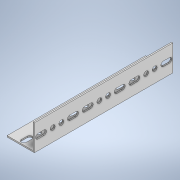
# Autodesk Inventor part: ChassisFrame
Saved by Autodesk Inventor 2020 (Build 240168000, 168)
## iProperties
Created: 2021-11-11
Part Number: ChassisFrame
Material: Generic
Document SubType Name: Modeling
Designer: 17185
Density: 1 g/cm^3
Appearance: Default
Author: 17185
Autodesk Inventor part; units mm, degrees
ref_plane "YZ Plane" through (0, 0, 0) normal (1, 0, 0) x (0, 1, 0)
ref_plane "XZ Plane" through (0, 0, 0) normal (0, 1, 0) x (-1, 0, 0)
ref_plane "XY Plane" through (0, 0, 0) normal (0, 0, 1) x (1, 0, 0)
sketch "Sketch1" plane through (0, 0, 0) normal (0, 1, 0) x (-1, 0, 0)
  line L0 (19.05, 101.6) -> (-19.05, 101.6)
  line L1 (-19.05, 101.6) -> (-19.05, -101.6)
  line L2 (-19.05, -101.6) -> (19.05, -101.6)
  line L3 (19.05, -101.6) -> (19.05, 101.6)
  line L4 (19.05, 101.6) -> (-19.05, -101.6) construction
  line L5 (-19.05, 101.6) -> (19.05, -101.6) construction
  circle A0 centre (0, 62.23) radius 3.556
  circle A1 centre (0, 6.35) radius 3.556
  line L6 (0, 101.6) -> (0, -101.6) construction
  line L7 (0, 49.53) -> (0, 40.64) construction
  line L8 (3.556, 49.53) -> (3.556, 40.64)
  line L9 (-3.556, 40.64) -> (-3.556, 49.53)
  arc A2 (3.556, 49.53) -> (-3.556, 49.53) centre (0, 49.53) ccw
  arc A3 (-3.556, 40.64) -> (3.556, 40.64) centre (0, 40.64) ccw
  line L10 (0, 27.94) -> (0, 19.05) construction
  line L11 (-3.556, 27.94) -> (-3.556, 19.05)
  line L12 (3.556, 19.05) -> (3.556, 27.94)
  arc A4 (3.556, 27.94) -> (-3.556, 27.94) centre (0, 27.94) ccw
  arc A5 (-3.556, 19.05) -> (3.556, 19.05) centre (0, 19.05) ccw
  line L13 (19.05, 68.58) -> (-6.1251, 68.58) construction
  line L14 (-6.1251, 68.58) -> (-19.05, 68.58) construction
  circle A6 centre (0, 74.93) radius 3.556
  circle A7 centre (0, 130.81) radius 3.556
  line L15 (0, 87.63) -> (0, 96.52) construction
  line L16 (3.556, 87.63) -> (3.556, 96.52)
  line L17 (-3.556, 96.52) -> (-3.556, 87.63)
  arc A8 (-3.556, 87.63) -> (3.556, 87.63) centre (0, 87.63) ccw
  arc A9 (3.556, 96.52) -> (-3.556, 96.52) centre (0, 96.52) ccw
  line L18 (0, 109.22) -> (0, 118.11) construction
  line L19 (-3.556, 109.22) -> (-3.556, 118.11)
  line L20 (3.556, 118.11) -> (3.556, 109.22)
  arc A10 (-3.556, 109.22) -> (3.556, 109.22) centre (0, 109.22) ccw
  arc A11 (3.556, 118.11) -> (-3.556, 118.11) centre (0, 118.11) ccw
  line L21 (19.05, 0) -> (-19.05, 0) construction
  circle A12 centre (0, -62.23) radius 3.556
  circle A13 centre (0, -6.35) radius 3.556
  line L22 (0, -49.53) -> (0, -40.64) construction
  line L23 (3.556, -49.53) -> (3.556, -40.64)
  line L24 (-3.556, -40.64) -> (-3.556, -49.53)
  arc A14 (-3.556, -49.53) -> (3.556, -49.53) centre (0, -49.53) ccw
  arc A15 (3.556, -40.64) -> (-3.556, -40.64) centre (0, -40.64) ccw
  line L25 (0, -27.94) -> (0, -19.05) construction
  line L26 (-3.556, -27.94) -> (-3.556, -19.05)
  line L27 (3.556, -19.05) -> (3.556, -27.94)
  arc A16 (-3.556, -27.94) -> (3.556, -27.94) centre (0, -27.94) ccw
  arc A17 (3.556, -19.05) -> (-3.556, -19.05) centre (0, -19.05) ccw
  line L28 (0, -109.22) -> (0, -118.11) construction
  line L29 (3.556, -118.11) -> (3.556, -109.22)
  arc A18 (3.556, -109.22) -> (-3.556, -109.22) centre (0, -109.22) ccw
  arc A19 (-3.556, -118.11) -> (3.556, -118.11) centre (0, -118.11) ccw
  circle A20 centre (0, -130.81) radius 3.556
  line L30 (-3.556, -109.22) -> (-3.556, -118.11)
  line L31 (0, -87.63) -> (0, -96.52) construction
  line L32 (-3.556, -96.52) -> (-3.556, -87.63)
  arc A21 (-3.556, -96.52) -> (3.556, -96.52) centre (0, -96.52) ccw
  arc A22 (3.556, -87.63) -> (-3.556, -87.63) centre (0, -87.63) ccw
  circle A23 centre (0, -74.93) radius 3.556
  line L33 (3.556, -87.63) -> (3.556, -96.52)
  line L34 (19.05, -137.16) -> (-19.05, -137.16) construction
  line L35 (19.05, 137.16) -> (-19.05, 137.16) construction
  circle A24 centre (0, 212.09) radius 3.556
  circle A25 centre (0, 267.97) radius 3.556
  line L36 (0, 224.79) -> (0, 233.68) construction
  line L37 (3.556, 224.79) -> (3.556, 233.68)
  line L38 (-3.556, 233.68) -> (-3.556, 224.79)
  arc A26 (-3.556, 224.79) -> (3.556, 224.79) centre (0, 224.79) ccw
  arc A27 (3.556, 233.68) -> (-3.556, 233.68) centre (0, 233.68) ccw
  line L39 (0, 246.38) -> (0, 255.27) construction
  line L40 (-3.556, 246.38) -> (-3.556, 255.27)
  line L41 (3.556, 255.27) -> (3.556, 246.38)
  arc A28 (-3.556, 246.38) -> (3.556, 246.38) centre (0, 246.38) ccw
  arc A29 (3.556, 255.27) -> (-3.556, 255.27) centre (0, 255.27) ccw
  line L42 (0, 165.1) -> (0, 156.21) construction
  line L43 (3.556, 156.21) -> (3.556, 165.1)
  arc A30 (3.556, 165.1) -> (-3.556, 165.1) centre (0, 165.1) ccw
  arc A31 (-3.556, 156.21) -> (3.556, 156.21) centre (0, 156.21) ccw
  circle A32 centre (0, 143.51) radius 3.556
  line L44 (-3.556, 165.1) -> (-3.556, 156.21)
  line L45 (0, 186.69) -> (0, 177.8) construction
  line L46 (-3.556, 177.8) -> (-3.556, 186.69)
  arc A33 (-3.556, 177.8) -> (3.556, 177.8) centre (0, 177.8) ccw
  arc A34 (3.556, 186.69) -> (-3.556, 186.69) centre (0, 186.69) ccw
  circle A35 centre (0, 199.39) radius 3.556
  line L47 (3.556, 186.69) -> (3.556, 177.8)
  arc A36 (3.556, 302.26) -> (-3.556, 302.26) centre (0, 302.26) ccw
  arc A37 (-3.556, 293.37) -> (3.556, 293.37) centre (0, 293.37) ccw
  circle A38 centre (0, 280.67) radius 3.556
  line L48 (-3.556, 302.26) -> (-3.556, 293.37)
  line L49 (3.556, 293.37) -> (3.556, 302.26)
  line L50 (0, 302.26) -> (0, 293.37) construction
  circle A39 centre (0, -280.67) radius 3.556
  line L51 (0, -302.26) -> (0, -293.37) construction
  line L52 (-3.556, -302.26) -> (-3.556, -293.37)
  line L53 (3.556, -293.37) -> (3.556, -302.26)
  arc A40 (-3.556, -302.26) -> (3.556, -302.26) centre (0, -302.26) ccw
  arc A41 (3.556, -293.37) -> (-3.556, -293.37) centre (0, -293.37) ccw
  line L54 (19.05, -274.32) -> (-19.05, -274.32) construction
  arc A42 (3.556, -246.38) -> (-3.556, -246.38) centre (0, -246.38) ccw
  arc A43 (-3.556, -255.27) -> (3.556, -255.27) centre (0, -255.27) ccw
  circle A44 centre (0, -267.97) radius 3.556
  line L55 (-3.556, -246.38) -> (-3.556, -255.27)
  line L56 (3.556, -255.27) -> (3.556, -246.38)
  line L57 (0, -246.38) -> (0, -255.27) construction
  line L58 (0, -224.79) -> (0, -233.68) construction
  line L59 (-3.556, -233.68) -> (-3.556, -224.79)
  circle A45 centre (0, -212.09) radius 3.556
  arc A46 (3.556, -224.79) -> (-3.556, -224.79) centre (0, -224.79) ccw
  line L60 (3.556, -224.79) -> (3.556, -233.68)
  arc A47 (-3.556, -233.68) -> (3.556, -233.68) centre (0, -233.68) ccw
  arc A48 (3.556, -177.8) -> (-3.556, -177.8) centre (0, -177.8) ccw
  arc A49 (-3.556, -165.1) -> (3.556, -165.1) centre (0, -165.1) ccw
  line L61 (0, -165.1) -> (0, -156.21) construction
  line L62 (-3.556, -165.1) -> (-3.556, -156.21)
  line L63 (3.556, -156.21) -> (3.556, -165.1)
  arc A50 (3.556, -156.21) -> (-3.556, -156.21) centre (0, -156.21) ccw
  circle A51 centre (0, -143.51) radius 3.556
  line L64 (0, -186.69) -> (0, -177.8) construction
  line L65 (-3.556, -177.8) -> (-3.556, -186.69)
  line L66 (3.556, -186.69) -> (3.556, -177.8)
  arc A52 (-3.556, -186.69) -> (3.556, -186.69) centre (0, -186.69) ccw
  circle A53 centre (0, -199.39) radius 3.556
  point P0 (0, 0)
  point P1 (0, 45.085)
  point P2 (0, 23.495)
  point P3 (0, 92.075)
  point P4 (0, 113.665)
  point P5 (0, -45.085)
  point P6 (0, -23.495)
  point P7 (-6.1251, -68.58)
  point P8 (0, -113.665)
  point P9 (0, -92.075)
  point P10 (0, 274.32)
  point P11 (0, 229.235)
  point P12 (0, 250.825)
  point P13 (-6.1251, 205.74)
  point P14 (0, 160.655)
  point P15 (0, 182.245)
  point P16 (0, 297.815)
  point P17 (0, -274.32)
  point P18 (0, -297.815)
  point P19 (0, -250.825)
  point P20 (0, -229.235)
  point P21 (0, -160.655)
  point P22 (-6.1251, -205.74)
  point P23 (0, -182.245)
  point P24 (2.4887, -304.8)
  point P25 (2.4887, 304.8)
  point P26 (-2.4887, 304.8)
  point P27 (-2.4887, -304.8)
  dimension "d1" = 203.2
  dimension "d3" = 7.112
  dimension "d6" = 7.112
  dimension "d9" = 3.556
  dimension "d10" = 3.556
  dimension "d11" = 6.35
  dimension "d12" = 12.7
  dimension "d13" = 8.89
  dimension "d14" = 8.89
  dimension "d15" = 12.7
  dimension "d16" = 12.7
  dimension "d26" = 6.35
  dimension "d29" = 6.35
  dimension "d30" = 6.35
  constraints: 170 end point, 135 symmetric about line, 72 point on circle, 54 centre point, 11 point on line, 8 midpoint, 8 tangent, 4 parallel, 3 perpendicular, 2 horizontal, 48 other
  measures "d1" distance of L0.end L1.end
  measures "d3" diameter of A1
  measures "d6" diameter of A0
  measures "d9" radius of A5
  measures "d10" radius of A3
  measures "d11" distance of A1.centre point (0, 0)
  measures "d12" distance of L10.end A1.centre
  measures "d13" distance of L10.start L10.end
  measures "d14" distance of L7.start L7.end
  measures "d15" distance of L10.start L7.end
  measures "d16" distance of L7.start A0.centre
  measures "d26" distance from line of A0.centre L13
  measures "d29" distance from line of L34 A20.centre
  measures "d30" distance from line of L35 A7.centre
extrude "Extrusion1" add sketch "Sketch1" along normal blind 1.9844 contours L3 L2 L1 L0
sketch "Sketch5" plane through (19.05, 0, 101.6) normal (1, 0, 0) x (0, 0, -1)
  line L0 (0.0028, 0.1675) -> (203.2028, 0.1675)
  line L1 (203.2028, 0.1675) -> (203.2028, 38.2675)
  line L2 (203.2028, 38.2675) -> (0.0028, 38.2675)
  line L3 (0.0028, 38.2675) -> (0.0028, 0.1675)
  line L4 (101.6, 0) -> (101.6028, 38.2675) construction
  line L5 (0.0028, 18.2829) -> (203.2028, 19.2175) construction
  circle A0 centre (95.2514, 18.721) radius 3.556
  line L6 (82.5514, 18.6626) -> (73.6615, 18.6217) construction
  line L7 (82.535, 22.2186) -> (73.6451, 22.1777)
  line L8 (73.6778, 15.0658) -> (82.5677, 15.1066)
  arc A1 (82.5677, 15.1066) -> (82.535, 22.2186) centre (82.5514, 18.6626) ccw
  arc A2 (73.6451, 22.1777) -> (73.6778, 15.0658) centre (73.6615, 18.6217) ccw
  line L9 (0, 0) -> (203.2, 0) construction
  line L10 (67.3115, 38.2675) -> (67.3115, 0) construction
  circle A3 centre (39.3716, 18.721) radius 3.556
  line L11 (52.0716, 18.6626) -> (60.9615, 18.6217) construction
  line L12 (52.0879, 22.2186) -> (60.9778, 22.1777)
  line L13 (60.9451, 15.0658) -> (52.0552, 15.1066)
  arc A4 (52.0879, 22.2186) -> (52.0552, 15.1066) centre (52.0716, 18.6626) ccw
  arc A5 (60.9451, 15.0658) -> (60.9778, 22.1777) centre (60.9615, 18.6217) ccw
  line L14 (33.0216, 38.2675) -> (33.0216, 0) construction
  circle A6 centre (-29.2082, 18.721) radius 3.556
  line L15 (-16.5082, 18.6626) -> (-7.6183, 18.6217) construction
  line L16 (-16.4919, 22.2186) -> (-7.602, 22.1777)
  line L17 (-7.6347, 15.0658) -> (-16.5246, 15.1066)
  arc A7 (-16.4919, 22.2186) -> (-16.5246, 15.1066) centre (-16.5082, 18.6626) ccw
  arc A8 (-7.6347, 15.0658) -> (-7.602, 22.1777) centre (-7.6183, 18.6217) ccw
  line L18 (13.9716, 18.6626) -> (5.0817, 18.6217) construction
  line L19 (5.098, 15.0658) -> (13.9879, 15.1066)
  arc A9 (5.0653, 22.1777) -> (5.098, 15.0658) centre (5.0817, 18.6217) ccw
  circle A10 centre (26.6716, 18.721) radius 3.556
  arc A11 (13.9879, 15.1066) -> (13.9552, 22.2186) centre (13.9716, 18.6626) ccw
  line L20 (13.9552, 22.2186) -> (5.0653, 22.1777)
  line L21 (-35.5582, 38.2675) -> (-35.5582, 0) construction
  circle A12 centre (-166.3679, 18.721) radius 3.556
  line L22 (-153.6679, 18.6626) -> (-144.778, 18.6217) construction
  line L23 (-153.6515, 22.2186) -> (-144.7616, 22.1777)
  line L24 (-144.7943, 15.0658) -> (-153.6842, 15.1066)
  arc A13 (-153.6515, 22.2186) -> (-153.6842, 15.1066) centre (-153.6679, 18.6626) ccw
  arc A14 (-144.7943, 15.0658) -> (-144.7616, 22.1777) centre (-144.778, 18.6217) ccw
  line L25 (-123.188, 18.6626) -> (-132.078, 18.6217) construction
  line L26 (-132.0616, 15.0658) -> (-123.1717, 15.1066)
  arc A15 (-132.0943, 22.1777) -> (-132.0616, 15.0658) centre (-132.078, 18.6217) ccw
  circle A16 centre (-110.488, 18.721) radius 3.556
  arc A17 (-123.1717, 15.1066) -> (-123.2044, 22.2186) centre (-123.188, 18.6626) ccw
  line L27 (-123.2044, 22.2186) -> (-132.0943, 22.1777)
  arc A18 (-85.0717, 22.2186) -> (-85.1044, 15.1066) centre (-85.088, 18.6626) ccw
  line L28 (-85.088, 18.6626) -> (-76.1981, 18.6217) construction
  line L29 (-85.0717, 22.2186) -> (-76.1818, 22.1777)
  arc A19 (-76.2145, 15.0658) -> (-76.1818, 22.1777) centre (-76.1981, 18.6217) ccw
  arc A20 (-63.5145, 22.1777) -> (-63.4818, 15.0658) centre (-63.4981, 18.6217) ccw
  line L30 (-54.6246, 22.2186) -> (-63.5145, 22.1777)
  line L31 (-63.4818, 15.0658) -> (-54.5919, 15.1066)
  arc A21 (-54.5919, 15.1066) -> (-54.6246, 22.2186) centre (-54.6082, 18.6626) ccw
  circle A22 centre (-41.9082, 18.721) radius 3.556
  circle A23 centre (-97.788, 18.721) radius 3.556
  line L32 (-54.6082, 18.6626) -> (-63.4981, 18.6217) construction
  line L33 (-76.2145, 15.0658) -> (-85.1044, 15.1066)
  line L34 (-172.7179, 38.2675) -> (-172.7179, 0) construction
  arc A24 (-191.7515, 15.1066) -> (-191.7842, 22.2186) centre (-191.7679, 18.6626) ccw
  line L35 (-191.7679, 18.6626) -> (-200.6578, 18.6217) construction
  line L36 (-200.6414, 15.0658) -> (-191.7515, 15.1066)
  arc A25 (-200.6741, 22.1777) -> (-200.6414, 15.0658) centre (-200.6578, 18.6217) ccw
  circle A26 centre (-179.0679, 18.721) radius 3.556
  line L37 (-191.7842, 22.2186) -> (-200.6741, 22.1777)
  circle A27 centre (107.9514, 18.7201) radius 3.556
  line L38 (120.6514, 18.6598) -> (129.5413, 18.6176) construction
  line L39 (120.6683, 22.2157) -> (129.5582, 22.1735)
  line L40 (129.5244, 15.0616) -> (120.6345, 15.1038)
  arc A28 (120.6683, 22.2157) -> (120.6345, 15.1038) centre (120.6514, 18.6598) ccw
  arc A29 (129.5244, 15.0616) -> (129.5582, 22.1735) centre (129.5413, 18.6176) ccw
  line L41 (151.1312, 18.6553) -> (142.2413, 18.6157) construction
  line L42 (142.2571, 15.0597) -> (151.147, 15.0993)
  arc A30 (142.2255, 22.1717) -> (142.2571, 15.0597) centre (142.2413, 18.6157) ccw
  circle A31 centre (163.8312, 18.7118) radius 3.556
  arc A32 (151.147, 15.0993) -> (151.1154, 22.2112) centre (151.1312, 18.6553) ccw
  line L43 (151.1154, 22.2112) -> (142.2255, 22.1717)
  arc A33 (189.2481, 22.2056) -> (189.2143, 15.0936) centre (189.2312, 18.6496) ccw
  line L44 (189.2312, 18.6496) -> (198.1211, 18.6074) construction
  line L45 (189.2481, 22.2056) -> (198.138, 22.1634)
  arc A34 (198.1042, 15.0514) -> (198.138, 22.1634) centre (198.1211, 18.6074) ccw
  arc A35 (210.8053, 22.1615) -> (210.8369, 15.0496) centre (210.8211, 18.6055) ccw
  line L46 (219.6952, 22.2011) -> (210.8053, 22.1615)
  line L47 (210.8369, 15.0496) -> (219.7268, 15.0891)
  arc A36 (219.7268, 15.0891) -> (219.6952, 22.2011) centre (219.711, 18.6451) ccw
  circle A37 centre (232.411, 18.7016) radius 3.556
  circle A38 centre (176.5312, 18.7099) radius 3.556
  line L48 (219.711, 18.6451) -> (210.8211, 18.6055) construction
  line L49 (198.1042, 15.0514) -> (189.2143, 15.0936)
  arc A39 (356.8865, 15.0688) -> (356.8548, 22.1807) centre (356.8706, 18.6247) ccw
  line L50 (356.8706, 18.6247) -> (347.9807, 18.5852) construction
  line L51 (347.9965, 15.0292) -> (356.8865, 15.0688)
  arc A40 (347.9649, 22.1411) -> (347.9965, 15.0292) centre (347.9807, 18.5852) ccw
  arc A41 (335.2638, 15.0311) -> (335.2976, 22.143) centre (335.2807, 18.5871) ccw
  line L52 (326.3908, 18.6293) -> (335.2807, 18.5871) construction
  arc A42 (326.4077, 22.1852) -> (326.3739, 15.0733) centre (326.3908, 18.6293) ccw
  circle A43 centre (369.5706, 18.6813) radius 3.556
  line L53 (356.8548, 22.1807) -> (347.9649, 22.1411)
  circle A44 centre (313.6908, 18.6896) radius 3.556
  line L54 (326.4077, 22.1852) -> (335.2976, 22.143)
  line L55 (335.2638, 15.0311) -> (326.3739, 15.0733)
  circle A45 centre (300.9908, 18.6914) radius 3.556
  arc A46 (288.3066, 15.079) -> (288.275, 22.1909) centre (288.2908, 18.6349) ccw
  line L56 (288.275, 22.1909) -> (279.3851, 22.1513)
  line L57 (288.2908, 18.6349) -> (279.4009, 18.5953) construction
  line L58 (279.4167, 15.0394) -> (288.3066, 15.079)
  arc A47 (279.3851, 22.1513) -> (279.4167, 15.0394) centre (279.4009, 18.5953) ccw
  arc A48 (266.684, 15.0413) -> (266.7178, 22.1532) centre (266.7009, 18.5972) ccw
  line L59 (257.8279, 22.1954) -> (266.7178, 22.1532)
  line L60 (257.811, 18.6394) -> (266.7009, 18.5972) construction
  line L61 (266.684, 15.0413) -> (257.7941, 15.0835)
  arc A49 (257.8279, 22.1954) -> (257.7941, 15.0835) centre (257.811, 18.6394) ccw
  circle A50 centre (245.111, 18.6997) radius 3.556
  arc A51 (394.9875, 22.1751) -> (394.9537, 15.0631) centre (394.9706, 18.6191) ccw
  line L62 (394.9706, 18.6191) -> (403.8605, 18.5769) construction
  line L63 (403.8436, 15.0209) -> (394.9537, 15.0631)
  arc A52 (403.8436, 15.0209) -> (403.8774, 22.1329) centre (403.8605, 18.5769) ccw
  line L64 (394.9875, 22.1751) -> (403.8774, 22.1329)
  circle A53 centre (382.2706, 18.6794) radius 3.556
  point P0 (78.1064, 18.6422)
  point P1 (56.5165, 18.6422)
  point P2 (-12.0633, 18.6422)
  point P3 (9.5266, 18.6422)
  point P4 (-149.2229, 18.6422)
  point P5 (-127.633, 18.6422)
  point P6 (-80.6431, 18.6422)
  point P7 (-59.0532, 18.6422)
  point P8 (-196.2128, 18.6422)
  point P9 (203.1999, 18.2679)
  point P10 (125.0963, 18.6387)
  point P11 (146.6862, 18.6355)
  point P12 (193.6761, 18.6285)
  point P13 (215.266, 18.6253)
  point P14 (352.4257, 18.605)
  point P15 (330.8358, 18.6082)
  point P16 (283.8459, 18.6151)
  point P17 (262.256, 18.6183)
  point P18 (399.4156, 18.598)
  point P19 (457.2028, 21.1288)
  point P20 (-152.3972, 21.1766)
  point P21 (-152.3972, 16.1965)
  point P22 (457.2028, 16.1547)
  dimension "d61" = 203.2
  dimension "d62" = 38.1
  dimension "d63" = 7.112
  dimension "d64" = 8.89
  dimension "d65" = 7.112
  dimension "d66" = 6.35
  dimension "d67" = 12.7
  dimension "d72" = 6.35
  dimension "d73" = 6.35
  dimension "d74" = 6.35
  dimension "d75" = 6.35
  constraints: 164 end point, 137 symmetric about line, 72 point on circle, 54 centre point, 12 point on line, 4 tangent, 3 midpoint, 3 parallel, 3 perpendicular, 2 vertical, 1 horizontal, 51 other
  measures "d61" distance of L2.end L1.end
  measures "d62" distance of L0.end L1.end
  measures "d63" diameter of A0
  measures "d64" distance of L6.start L6.end
  measures "d65" diameter of A2
  measures "d66" distance from line of L4 A0.centre
  measures "d67" horizontal distance of A0.centre L6.start
  measures "d72" distance from line of L10 L6.end
  measures "d73" distance from line of L14 A3.centre
  measures "d74" distance from line of L21 A6.centre
  measures "d75" distance from line of L34 A12.centre
extrude "Extrusion2" add sketch "Sketch5" along normal blind 1.9844 contours L3 L2 L1 L0
equation "\"d6\" = d3"
equation "\"d9\" = 0.5 * d3"
equation "\"d10\" = d9"
equation "\"d14\" = d13"
equation "\"d15\" = d12"
equation "\"d16\" = d12"
equation "\"d65\" = d63"
equation "\"d72\" = d66"
equation "\"d73\" = d66"
equation "\"d74\" = d66"
equation "\"d75\" = d66"
body "Solid1"
